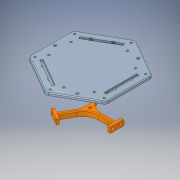
# Autodesk Inventor part: Stewart-Platform-Base-Innen
Saved by Autodesk Inventor 2018.2 (Build 222227000, 227)
## iProperties
Created: 2018-02-17
Part Number: Stewart-Platform-Base-Innen
Material: Generisch
Document SubType Name: Modeling
Designer: JochenAlt
Density: 1 g/cm^3
Appearance: Vorgabe
Author: JochenAlt
Autodesk Inventor part; units mm, degrees
ref_plane "YZ Plane" through (0, 0, 0) normal (1, 0, 0) x (0, 1, 0)
ref_plane "XZ Plane" through (0, 0, 0) normal (0, 1, 0) x (-1, 0, 0)
sketch "Skizze1" plane through (0, 0, 0) normal (0, 0, 1) x (1, 0, 0)
  line L0 (0, 77.2198) -> (0, -77.2198) construction
  line L1 (-68.9409, 0) -> (68.4148, 0) construction
  line L2 (30.6, 28.85) -> (43.1, 28.85) construction
  line L3 (46.4, 25.55) -> (46.4, -25.55) construction
  line L4 (43.1, -28.85) -> (30.6, -28.85) construction
  line L5 (27.3, -25.55) -> (27.3, 25.55) construction
  arc A0 (30.6, 28.85) -> (27.3, 25.55) centre (30.6, 25.55) ccw construction
  arc A1 (46.4, 25.55) -> (43.1, 28.85) centre (43.1, 25.55) ccw construction
  arc A2 (43.1, -28.85) -> (46.4, -25.55) centre (43.1, -25.55) ccw construction
  arc A3 (27.3, -25.55) -> (30.6, -28.85) centre (30.6, -25.55) ccw construction
  circle A4 centre (30.6, 25.55) radius 1.25
  circle A5 centre (43.1, 25.55) radius 1.25
  circle A6 centre (30.6, -25.55) radius 1.25
  circle A7 centre (43.1, -25.55) radius 1.25
  line L6 (40.4, 20.25) -> (40.4, -20.25)
  line L7 (37.3, 20.25) -> (37.3, -20.25)
  line L8 (37.3, 20.25) -> (40.4, 20.25)
  line L9 (37.3, -20.25) -> (40.4, -20.25)
  line L10 (37.3, 0.8) -> (40.4, 0.8)
  line L11 (37.3, -0.8) -> (40.4, -0.8)
  line L12 (40.4, 11.55) -> (43.416, 11.55)
  line L13 (43.416, 11.55) -> (43.416, 8.75)
  line L14 (43.416, 8.75) -> (40.4, 8.75)
  line L15 (40.4, -8.75) -> (43.416, -8.75)
  line L16 (43.416, -8.75) -> (43.416, -11.55)
  line L17 (43.416, -11.55) -> (40.4, -11.55)
  line L18 (43.1, 29.15) -> (30.6, 29.15)
  arc A8 (30.6, 29.15) -> (27, 25.55) centre (30.6, 25.55) ccw
  line L19 (27, 25.55) -> (27, -25.55)
  arc A9 (27, -25.55) -> (30.6, -29.15) centre (30.6, -25.55) ccw
  line L20 (30.6, -29.15) -> (43.1, -29.15)
  arc A10 (43.1, -29.15) -> (46.7, -25.55) centre (43.1, -25.55) ccw
  line L21 (46.7, -25.55) -> (46.7, 25.55)
  arc A11 (46.7, 25.55) -> (43.1, 29.15) centre (43.1, 25.55) ccw
  line L22 (24.9713, -28.9965) -> (27.5298, -27.4299) construction
  line L23 (48.7, 0) -> (46.7, 0) construction
  circle A12 centre (0, 0) radius 48.7 construction
  line L24 (34.7269, 29.3354) -> (33.253, 27.9834) construction
  line L25 (46.7, -19.95) -> (40.4, -19.95)
  line L26 (46.7, 19.95) -> (40.4, 19.95)
  arc A13 (3.6946, 51.9007) -> (-1.2231, 53.2184) centre (0.5769, 50.1007) ccw
  circle A14 centre (0.5769, 50.1007) radius 1.25
  line L27 (-1.2231, 53.2184) -> (-45.4769, 27.6684)
  line L28 (-6.0728, 50.4184) -> (-2.9228, 44.9624)
  line L29 (-11.7054, 43.3744) -> (-10.1974, 40.7624)
  line L30 (-14.1303, 41.9744) -> (-11.7054, 43.3744)
  line L31 (-12.6223, 39.3624) -> (-14.1303, 41.9744)
  line L32 (-37.737, 24.8624) -> (-2.663, 45.1124)
  line L33 (-1.113, 42.4277) -> (-2.663, 45.1124)
  line L34 (-36.187, 22.1777) -> (-1.113, 42.4277)
  line L35 (-17.9572, 32.7027) -> (-19.5072, 35.3874)
  line L36 (-19.3428, 31.9027) -> (-20.8928, 34.5874)
  line L37 (-31.7106, 31.8244) -> (-29.2857, 33.2244)
  line L38 (-29.2857, 33.2244) -> (-27.7777, 30.6124)
  line L39 (-30.2026, 29.2124) -> (-31.7106, 31.8244)
  line L40 (-40.6272, 30.4684) -> (-37.4772, 25.0124)
  line L41 (-36.187, 22.1777) -> (-37.737, 24.8624)
  arc A15 (-45.4769, 27.6684) -> (-46.7946, 22.7507) centre (-43.6769, 24.5507) ccw
  circle A16 centre (-43.6769, 24.5507) radius 1.25
  line L42 (-46.7946, 22.7507) -> (-40.5446, 11.9254)
  circle A17 centre (6.8269, 39.2754) radius 1.25
  arc A18 (8.6269, 36.1577) -> (9.9446, 41.0754) centre (6.8269, 39.2754) ccw
  line L43 (-35.6269, 10.6077) -> (8.6269, 36.1577)
  circle A19 centre (-37.4269, 13.7254) radius 1.25
  arc A20 (-40.5446, 11.9254) -> (-35.6269, 10.6077) centre (-37.4269, 13.7254) ccw
  line L44 (9.9446, 41.0754) -> (3.6946, 51.9007)
  arc A21 (-46.7946, -22.7507) -> (-45.4769, -27.6684) centre (-43.6769, -24.5507) ccw
  circle A22 centre (-43.6769, -24.5507) radius 1.25
  line L45 (-45.4769, -27.6684) -> (-1.2231, -53.2184)
  line L46 (-40.6272, -30.4684) -> (-37.4772, -25.0124)
  line L47 (-31.7106, -31.8244) -> (-30.2026, -29.2124)
  line L48 (-29.2857, -33.2244) -> (-31.7106, -31.8244)
  line L49 (-27.7777, -30.6124) -> (-29.2857, -33.2244)
  line L50 (-2.663, -45.1124) -> (-37.737, -24.8624)
  line L51 (-36.187, -22.1777) -> (-37.737, -24.8624)
  line L52 (-1.113, -42.4277) -> (-36.187, -22.1777)
  line L53 (-19.3428, -31.9027) -> (-20.8928, -34.5874)
  line L54 (-17.9572, -32.7027) -> (-19.5072, -35.3874)
  line L55 (-11.7054, -43.3744) -> (-14.1303, -41.9744)
  line L56 (-14.1303, -41.9744) -> (-12.6223, -39.3624)
  line L57 (-10.1974, -40.7624) -> (-11.7054, -43.3744)
  line L58 (-6.0728, -50.4184) -> (-2.9228, -44.9624)
  line L59 (-1.113, -42.4277) -> (-2.663, -45.1124)
  arc A23 (-1.2231, -53.2184) -> (3.6946, -51.9007) centre (0.5769, -50.1007) ccw
  circle A24 centre (0.5769, -50.1007) radius 1.25
  line L60 (3.6946, -51.9007) -> (9.9446, -41.0754)
  circle A25 centre (-37.4269, -13.7254) radius 1.25
  arc A26 (-35.6269, -10.6077) -> (-40.5446, -11.9254) centre (-37.4269, -13.7254) ccw
  line L61 (8.6269, -36.1577) -> (-35.6269, -10.6077)
  circle A27 centre (6.8269, -39.2754) radius 1.25
  arc A28 (9.9446, -41.0754) -> (8.6269, -36.1577) centre (6.8269, -39.2754) ccw
  line L62 (-40.5446, -11.9254) -> (-46.7946, -22.7507)
  line L63 (47.4871, -28.1507) -> (46.1968, -27.3858) construction
  line L64 (48.2, -25.55) -> (48.2, 25.55)
  line L65 (-1.9506, -54.4786) -> (-46.2045, -28.9286)
  line L66 (-46.2045, 28.9286) -> (-1.9506, 54.4786)
  arc A29 (-46.2045, 28.9286) -> (-48.7321, 24.5507) centre (-43.6769, 24.5507) ccw
  line L67 (3.1005, 54.4809) -> (45.646, 29.9691)
  line L68 (-48.7321, -24.5507) -> (-48.7321, 24.5507)
  arc A30 (3.1005, 54.4809) -> (-1.9506, 54.4786) centre (0.5769, 50.1007) ccw
  arc A31 (48.2, 25.55) -> (45.646, 29.9691) centre (43.1, 25.55) ccw
  arc A32 (40.2364, 29.15) -> (40.1916, 29.1139) centre (43.1, 25.55) ccw
  arc A33 (45.646, -29.9691) -> (48.2, -25.55) centre (43.1, -25.55) ccw
  line L69 (45.646, -29.9691) -> (3.1005, -54.4809)
  arc A34 (-1.9506, -54.4786) -> (3.1005, -54.4809) centre (0.5769, -50.1007) ccw
  arc A35 (-48.7321, -24.5507) -> (-46.2045, -28.9286) centre (-43.6769, -24.5507) ccw
  circle A36 centre (0, 0) radius 43.5 construction
  circle A37 centre (-43.5, 0) radius 1.65
  circle A38 centre (21.75, -37.6721) radius 1.65
  circle A39 centre (21.75, 37.6721) radius 1.65
  line L70 (21.75, -37.6721) -> (0, 0) construction
  line L71 (0, 0) -> (21.75, 37.6721) construction
  point P0 (43.416, -10.15)
  point P1 (0, 0)
  point P2 (46.7, -21.4)
  point P3 (46.7, 21.4)
  point P4 (-23.35, 40.4434)
  point P5 (-4.8171, 51.1434)
  point P6 (-41.8829, 29.7434)
  point P7 (-12.9178, 42.6744)
  point P8 (9.9901, 37.5565)
  point P9 (-40.8609, 14.8062)
  point P10 (-23.35, -40.4434)
  point P11 (-41.8829, -29.7434)
  point P12 (-4.8171, -51.1434)
  point P13 (-30.4982, -32.5244)
  point P14 (-37.5199, -10.1266)
  point P15 (7.6079, -42.7897)
  dimension "d1" = 57.7
  dimension "d2" = 19.1
  dimension "d3" = 3.3
  dimension "d5" = 2.5
  dimension "d6" = 6
  dimension "d7" = 3.1
  dimension "d9" = 1.6
  dimension "d10" = 2.984
  dimension "d11" = 2.8
  dimension "d12" = 17.5
  dimension "d21" = 0.3
  dimension "d22" = 3
  dimension "d34" = 2
  dimension "d35" = 2
  dimension "d105" = 360
  dimension "d107" = 40.5
  dimension "d108" = 0.3
  dimension "d140" = 1.5
  dimension "d141" = 27
  dimension "d145" = 1.5
  dimension "d148" = 87
  dimension "d149" = 3.3
  dimension "d150" = 120
  constraints: 134 end point, 56 point on circle, 39 centre point, 23 point on line, 21 coincident, 20 tangent, 10 horizontal, 8 equal radius, 7 parallel, 5 midpoint, 5 perpendicular, 3 line through centre, 1 collinear, 1 horizontal alignment, 1 symmetric about line, 1 vertical, 253 other
  measures "d1" distance between parallel lines of L4 L2
  measures "d2" distance between parallel lines of L3 L5
  measures "d3" radius of A0
  measures "d5" diameter of A4
  measures "d9" distance between parallel lines of L11 L10
  measures "d10" distance between parallel lines of L3 L13
  measures "d11" distance between parallel lines of L14 L12
  measures "d12" distance between parallel lines of L15 L14
  measures "d21" distance between parallel lines of L19 L5
  measures "d22" distance of L22.end L22.start
  measures "d34" distance of L23.start L23.end
  measures "d35" distance of L24.start L24.end
  measures "d107" distance between parallel lines of L8 L9
  measures "d108" distance between parallel lines of L25 L9
  measures "d140" distance of L63.start L63.end
  measures "d141" distance between parallel lines of L0 L19
  measures "d145" distance between parallel lines of L21 L64
  measures "d148" diameter of A36
  measures "d149" diameter of A37
  measures "d150" angle of L71 L70
extrude "Extrusion5" add sketch "Skizze1" along normal blind 4 contours L8 L7 L9 L6 L25 L21 A10 L20 A9 L19 A8 L18 A11 L26 | L26 L21 L25 L6 L17 L16 L15 L14 L13 L12 | L44 A18 L43 A20 L42 A15 L27 L40 L32 L41 L34 L33 L28 A13 | L28 L32 L29 L30 L31 L38 L37 L39 L40 L27 | L62 A26 L61 A28 L60 A23 L45 L58 L50 L59 L52 L51 L46 A21 | L46 L50 L47 L48 L49 L56 L55 L57 L58 L45 | A33 L69 A34 L65 A35 L68 A29 L66 A30 L67 A31 L64
extrude "Extrusion4" cut sketch "Skizze1" along normal blind 2 contours L8 L7 L9 L6 L25 L21 A10 L20 A9 L19 A8 L18 A11 L26 | L12 L13 L14 L6 | L6 L15 L16 L17 | L44 A18 L43 A20 L42 A15 L27 L40 L32 L41 L34 L33 L28 A13 | L62 A26 L61 A28 L60 A23 L45 L58 L50 L59 L52 L51 L46 A21
ref_plane "Arbeitsebene2" through (0, 0, -40.8) normal (0, 0, 1) x (1, 0, 0)
sketch "Skizze6" plane through (0, 0, -40.8) normal (0, 0, 1) x (1, 0, 0)
  line L0 (40.4, -11.55) -> (40.4, -20.25) construction
  line L1 (40.4, -20.25) -> (37.3, -20.25) construction
  line L2 (37.3, -20.25) -> (37.3, 20.25) construction
  line L3 (40.4, 20.25) -> (40.4, 11.55) construction
  line L4 (37.3, 20.25) -> (40.4, 20.25) construction
  circle A0 centre (43.1, -25.55) radius 1.25 construction
  circle A1 centre (30.6, -25.55) radius 1.25 construction
  circle A2 centre (43.1, 25.55) radius 1.25 construction
  circle A3 centre (30.6, 25.55) radius 1.25 construction
  line L5 (33.1, 8.75) -> (33.1, -8.75)
  line L6 (33.1, 8.75) -> (30.1, 8.75)
  line L7 (40.4, -8.75) -> (40.4, 8.75) projected
  line L8 (-66.2313, 0) -> (62.7802, 0) construction
  line L9 (0, 37.52) -> (0, -37.52) construction
  line L10 (30.1, -8.75) -> (30.1, -2)
  line L11 (30.1, 2) -> (30.1, 8.75)
  line L12 (0, 0) -> (8.9019, 15.4186) construction
  line L13 (0, 0) -> (9.1171, -15.7912) construction
  arc A4 (2.7017, 4.6795) -> (12.7017, 2) centre (12.7017, 22) ccw
  arc A5 (12.7017, -2) -> (2.7017, -4.6795) centre (12.7017, -22) ccw
  line L14 (2.7017, 4.6795) -> (0, 6.2393)
  line L15 (2.7017, -4.6795) -> (0, -6.2393)
  line L16 (30.1, 2) -> (12.7017, 2)
  line L17 (30.1, -2) -> (12.7017, -2)
  line L18 (30.1, 8.75) -> (33.1, 8.75) projected
  line L19 (33.1, -8.75) -> (30.1, -8.75)
  arc A6 (0, -1.65) -> (0, 1.65) centre (0, 0) ccw
  line L20 (0, 6.2393) -> (0, 1.65)
  line L21 (0, -1.65) -> (0, -6.2393)
  line L22 (40.4, 8.75) -> (40.4, -8.75) projected
  line L23 (40.4, -8.75) -> (43.416, -8.75) projected
  line L24 (43.416, -8.75) -> (43.416, -11.55) projected
  line L25 (43.416, -11.55) -> (40.4, -11.55) projected
  line L26 (40.4, 11.55) -> (43.416, 11.55) projected
  line L27 (43.416, 11.55) -> (43.416, 8.75) projected
  line L28 (43.416, 8.75) -> (40.4, 8.75) projected
  point P0 (-47.8011, -0.8)
  dimension "d73" = 120
  dimension "d89" = 20
  dimension "d90" = 4
  dimension "d91" = 3.3
  dimension "d146" = 3
  dimension "d147" = 4.2
  constraints: 26 end point, 6 point on circle, 4 perpendicular, 4 point on line, 4 tangent, 3 centre point, 2 parallel, 1 coincident, 1 collinear, 1 other
  measures "d73" angle of L13 L12
  measures "d89" radius of A5
  measures "d90" distance between parallel lines of L16 L17
  measures "d91" diameter of A6
  measures "d146" distance between parallel lines of L11 L5
  measures "d147" distance between parallel lines of L5 L2
extrude "Extrusion9" add sketch "Skizze6" against normal blind 7.1 separate body
sketch "Skizze7" plane through (33.1, 8.75, -40.8) normal (1, 0, 0) x (0, 0, -1)
  circle A0 centre (3.8, -3.7) radius 1.7
  circle A1 centre (3.8, -13.8) radius 1.7
  line L0 (0, -17.5) -> (0, 0) construction
  line L1 (0, -8.75) -> (7.1, -8.75) construction
  line L2 (7.1, 0) -> (7.1, -17.5) construction
  point P0 (-40.8, -8.75)
  dimension "d76" = 3.4
  dimension "d77" = 10.1
  dimension "d88" = 3.3
  constraints: 2 centre point, 2 end point, 2 midpoint, 1 equal radius, 1 symmetric about line
  measures "d76" diameter of A1
  measures "d77" distance of A0.centre A1.centre
  measures "d88" distance from line of A0.centre L2
extrude "Extrusion10" cut sketch "Skizze7" against normal blind 10 bodies 1 2
pattern_circular "Runde Anordnung5" count 3 over 360 about axis through (0, 0, -10) along (0, 0, 1) of "Extrusion10", "Extrusion9" bodies 2
fillet "Rundung1" radius 1 30 edges at (2.7017, 4.6795, -40.8) (21.4009, 2, -40.8) (-8.9684, 19.5337, -40.8) (2.7017, -4.6795, -40.8) (-8.9684, -19.5337, -40.8) (21.4009, -2, -40.8) (-12.4325, -17.5337, -40.8) (-12.4325, 17.5337, -40.8) (-5.4034, 0, -40.8) (2.7017, 4.6795, -47.9) (21.4009, 2, -47.9) (-8.9684, 19.5337, -47.9) (-12.4325, 17.5337, -47.9) (-12.4325, -17.5337, -47.9) (-5.4034, 0, -47.9) (31.6, -8.75, -47.9) (31.6, 8.75, -47.9) (-8.2223, -31.7414, -47.9) (-23.3777, -22.9914, -47.9) (-23.3777, -22.9914, -40.8) (-8.2223, -31.7414, -40.8) (31.6, -8.75, -40.8) (31.6, 8.75, -40.8) (-8.2223, 31.7414, -40.8) (-8.2223, 31.7414, -47.9) (-23.3777, 22.9914, -40.8) (-23.3777, 22.9914, -47.9) (-8.9684, -19.5337, -47.9) (21.4009, -2, -47.9) (2.7017, -4.6795, -47.9)
fillet "Rundung2" radius 1 15 edges at (-24.0776, -41.7036, 4) (48.2, 0, 4) (-24.0776, 41.7036, 4) (47.5156, -28.102, 0) (48.2, 0, 0) (47.5156, 28.102, 0) (24.3732, 42.225, 0) (0.5746, 55.1559, 0) (-24.0776, 41.7036, 0) (-48.0548, 27.0783, 0) (-48.7321, 0, 0) (-48.0548, -27.0783, 0) (-24.0776, -41.7036, 0) (0.5746, -55.1559, 0) (24.3732, -42.225, 0)
sketch "Skizze8" plane through (0, 0, 4) normal (0, 0, 1) x (1, 0, 0)
  circle A0 centre (6.8269, -39.2754) radius 1.25 construction
  circle A1 centre (-37.4269, -13.7254) radius 1.25 construction
  circle A2 centre (0.5769, -50.1007) radius 1.25 construction
  circle A3 centre (-43.6769, -24.5507) radius 1.25 construction
  circle A4 centre (-37.4269, 13.7254) radius 1.25 construction
  circle A5 centre (6.8269, 39.2754) radius 1.25 construction
  circle A6 centre (-43.6769, 24.5507) radius 1.25 construction
  circle A7 centre (0.5769, 50.1007) radius 1.25 construction
  circle A8 centre (43.1, -25.55) radius 1.25 construction
  circle A9 centre (30.6, -25.55) radius 1.25 construction
  circle A10 centre (43.1, 25.55) radius 1.25 construction
  circle A11 centre (30.6, 25.55) radius 1.25 construction
  line L0 (-12.6223, -39.3624) -> (-27.7777, -30.6124) construction
  line L1 (-30.2026, -29.2124) -> (-37.737, -24.8624) construction
  line L2 (-37.737, -24.8624) -> (-36.187, -22.1777) construction
  line L3 (-36.187, -22.1777) -> (-1.113, -42.4277) construction
  line L4 (-1.113, -42.4277) -> (-2.663, -45.1124) construction
  line L5 (-27.7777, 30.6124) -> (-12.6223, 39.3624) construction
  line L6 (-10.1974, 40.7624) -> (-2.663, 45.1124) construction
  line L7 (-2.663, 45.1124) -> (-1.113, 42.4277) construction
  line L8 (-1.113, 42.4277) -> (-36.187, 22.1777) construction
  line L9 (-36.187, 22.1777) -> (-37.737, 24.8624) construction
  line L10 (40.4, 20.25) -> (40.4, 11.55) construction
  line L11 (37.3, -20.25) -> (37.3, 20.25) construction
  line L12 (37.3, 20.25) -> (40.4, 20.25) construction
  line L13 (40.4, -11.55) -> (40.4, -20.25) construction
  line L14 (40.4, -20.25) -> (37.3, -20.25) construction
  line L15 (40.4, -11.55) -> (43.416, -11.55) projected
  line L16 (40.4, 8.75) -> (43.416, 8.75) projected
  line L17 (43.416, 11.55) -> (40.4, 11.55) projected
  line L18 (41.216, 8.75) -> (43.416, 8.75)
  line L19 (43.416, 8.75) -> (43.416, 11.55)
  line L20 (43.416, 11.55) -> (41.216, 11.55)
  line L21 (41.216, 11.55) -> (41.216, 8.75)
  line L22 (-29.2857, -33.2244) -> (-27.7777, -30.6124) projected
  line L23 (-28.1857, -31.3191) -> (-13.0303, -40.0691) construction
  line L24 (-28.1857, 31.3191) -> (-13.0303, 40.0691) construction
  line L25 (-12.6223, 39.3624) -> (-14.1303, 41.9744) construction
  line L26 (-29.2857, 33.2244) -> (-27.7777, 30.6124) projected
  line L27 (-28.1857, 31.3191) -> (-29.2857, 33.2244)
  line L28 (-29.2857, 33.2244) -> (-31.7106, 31.8244)
  line L29 (-31.7106, 31.8244) -> (-30.6106, 29.9191)
  line L30 (-30.6106, 29.9191) -> (-28.1857, 31.3191)
  line L31 (-13.0303, 40.0691) -> (-14.1303, 41.9744)
  line L32 (-14.1303, 41.9744) -> (-11.7054, 43.3744)
  line L33 (-11.7054, 43.3744) -> (-10.6054, 41.4691)
  line L34 (-10.6054, 41.4691) -> (-13.0303, 40.0691)
  line L35 (-13.0303, -40.0691) -> (-14.1303, -41.9744)
  line L36 (-14.1303, -41.9744) -> (-11.7054, -43.3744)
  line L37 (-11.7054, -43.3744) -> (-10.6054, -41.4691)
  line L38 (-10.6054, -41.4691) -> (-13.0303, -40.0691)
  line L39 (-28.1857, -31.3191) -> (-29.2857, -33.2244)
  line L40 (-29.2857, -33.2244) -> (-31.7106, -31.8244)
  line L41 (-31.7106, -31.8244) -> (-30.6106, -29.9191)
  line L42 (-30.6106, -29.9191) -> (-28.1857, -31.3191)
  line L43 (-12.6223, 39.3624) -> (-14.1303, 41.9744) projected
  line L44 (-14.1303, 41.9744) -> (-11.7054, 43.3744) projected
  line L45 (-11.7054, 43.3744) -> (-10.1974, 40.7624) projected
  line L46 (-37.737, 24.8624) -> (-30.2026, 29.2124) projected
  line L47 (-30.2026, 29.2124) -> (-31.7106, 31.8244) projected
  line L48 (-31.7106, 31.8244) -> (-29.2857, 33.2244) projected
  line L49 (-29.2857, 33.2244) -> (-27.7777, 30.6124) projected
  line L50 (40.4, 8.75) -> (40.4, -8.75) projected
  line L51 (40.4, -8.75) -> (43.416, -8.75) projected
  line L52 (43.416, -8.75) -> (43.416, -11.55) projected
  line L53 (43.416, -11.55) -> (40.4, -11.55) projected
  line L54 (40.4, 11.55) -> (43.416, 11.55) projected
  line L55 (43.416, 11.55) -> (43.416, 8.75) projected
  line L56 (43.416, 8.75) -> (40.4, 8.75) projected
  line L57 (-2.663, -45.1124) -> (-10.1974, -40.7624) projected
  line L58 (-10.1974, -40.7624) -> (-11.7054, -43.3744) projected
  line L59 (-11.7054, -43.3744) -> (-14.1303, -41.9744) projected
  line L60 (-14.1303, -41.9744) -> (-12.6223, -39.3624) projected
  line L61 (-27.7777, -30.6124) -> (-29.2857, -33.2244) projected
  line L62 (-29.2857, -33.2244) -> (-31.7106, -31.8244) projected
  line L63 (-31.7106, -31.8244) -> (-30.2026, -29.2124) projected
  arc A12 (43.1, -29.15) -> (46.7, -25.55) centre (43.1, -25.55) ccw construction
  line L64 (46.7, -19.95) -> (40.4, -19.95) construction
  line L65 (40.4, -19.95) -> (40.4, -11.55) construction
  line L66 (40.4, -11.55) -> (43.416, -11.55) construction
  line L67 (43.416, -11.55) -> (43.416, -8.75) construction
  line L68 (43.416, -8.75) -> (40.4, -8.75) construction
  line L69 (40.4, -8.75) -> (40.4, 8.75) construction
  line L70 (40.4, 8.75) -> (43.416, 8.75) construction
  line L71 (43.416, 8.75) -> (43.416, 11.55) construction
  line L72 (43.416, 11.55) -> (40.4, 11.55) construction
  line L73 (40.4, 11.55) -> (40.4, 19.95) construction
  line L74 (40.4, 19.95) -> (46.7, 19.95) construction
  arc A13 (46.7, 25.55) -> (43.1, 29.15) centre (43.1, 25.55) ccw construction
  circle A14 centre (43.1, -25.55) radius 1.25 construction
  circle A15 centre (30.6, -25.55) radius 1.25 construction
  circle A16 centre (43.1, 25.55) radius 1.25 construction
  circle A17 centre (30.6, 25.55) radius 1.25 construction
  line L75 (40.4, 20.25) -> (40.4, 19.95) construction
  line L76 (37.3, 20.25) -> (40.4, 20.25) construction
  line L77 (37.3, -20.25) -> (37.3, 20.25) construction
  line L78 (40.4, -20.25) -> (37.3, -20.25) construction
  line L79 (40.4, -19.95) -> (40.4, -20.25) construction
  line L80 (46.7, -19.95) -> (40.4, -19.95) construction
  line L81 (46.7, -25.55) -> (46.7, -19.95) construction
  arc A18 (43.1, -29.15) -> (46.7, -25.55) centre (43.1, -25.55) ccw construction
  line L82 (30.6, -29.15) -> (43.1, -29.15) construction
  arc A19 (27, -25.55) -> (30.6, -29.15) centre (30.6, -25.55) ccw construction
  line L83 (27, 25.55) -> (27, -25.55) construction
  arc A20 (30.6, 29.15) -> (27, 25.55) centre (30.6, 25.55) ccw construction
  line L84 (43.1, 29.15) -> (30.6, 29.15) construction
  arc A21 (46.7, 25.55) -> (43.1, 29.15) centre (43.1, 25.55) ccw construction
  line L85 (46.7, 19.95) -> (46.7, 25.55) construction
  line L86 (40.4, 19.95) -> (46.7, 19.95) construction
  line L87 (43.416, -8.75) -> (40.4, -8.75) projected
  line L88 (43.416, -8.75) -> (41.216, -8.75)
  line L89 (41.216, -8.75) -> (41.216, -11.55)
  line L90 (41.216, -11.55) -> (43.416, -11.55)
  line L91 (43.416, -11.55) -> (43.416, -8.75)
  line L92 (41.216, 8.75) -> (41.216, -8.75) construction
  line L93 (40.4, -8.75) -> (43.416, -8.75) construction
  line L94 (46.7, 19.95) -> (46.7, 25.55) projected
  line L95 (43.1, 29.15) -> (30.6, 29.15) projected
  arc A22 (30.6, 29.15) -> (27, 25.55) centre (30.6, 25.55) ccw projected
  line L96 (27, 25.55) -> (27, -25.55) projected
  arc A23 (27, -25.55) -> (30.6, -29.15) centre (30.6, -25.55) ccw projected
  line L97 (30.6, -29.15) -> (43.1, -29.15) projected
  line L98 (46.7, -25.55) -> (46.7, -19.95) projected
  point P0 (0, 0)
  dimension "d142" = 0.816
  dimension "d144" = 0.816
  constraints: 54 end point, 13 parallel, 7 perpendicular, 4 point on line, 2 collinear, 1 horizontal
  measures "d142" distance between parallel lines of L5 L24
  measures "d144" distance between parallel lines of L50 L92
extrude "Extrusion11" add sketch "Skizze8" against normal blind 4 bodies 1
chamfer "Fase3" distance 2 distance2 4 1 edges at (-11.8178, -40.7691, 0) measured on face at (-12.0678, -41.2021, 0)
chamfer "Fase4" distance 2 distance2 4 1 edges at (-29.3982, -30.6191, 0) measured on face at (-29.6482, -31.0521, 0)
chamfer "Fase5" distance 2 distance2 4 1 edges at (-11.8178, 40.7691, 0) measured on face at (-12.0678, 41.2021, 0)
chamfer "Fase6" distance 2 distance2 4 1 edges at (-29.3982, 30.6191, 0) measured on face at (-29.6482, 31.0521, 0)
chamfer "Fase7" distance 2 distance2 4 1 edges at (41.216, -10.15, 0) measured on face at (41.716, -10.15, 0)
chamfer "Fase8" distance 2 distance2 4 1 edges at (41.216, 10.15, 0) measured on face at (41.716, 10.15, 0)
equation "\"d22\" = d20"
equation "\"d35\" = d34"
equation "\"d44\" = d21"
equation "\"d20\" = 3"
